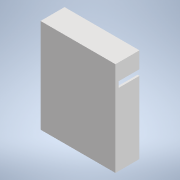
# Autodesk Inventor part: btn
Saved by Autodesk Inventor 2022 (Build 260153000, 153)
## iProperties
Created: 2025-06-23
Part Number: btn
Material: Типовые
Document SubType Name: Modeling
Designer: korsh524
Density: 1 g/cm^3
Appearance: По умолчанию
Author: korsh524
Autodesk Inventor part; units mm, degrees
ref_plane "YZ Plane" through (0, 0, 0) normal (1, 0, 0) x (0, 1, 0)
ref_plane "XZ Plane" through (0, 0, 0) normal (0, 1, 0) x (-1, 0, 0)
ref_plane "XY Plane" through (0, 0, 0) normal (0, 0, 1) x (1, 0, 0)
sketch "Эскиз1" plane through (0, 0, 0) normal (0, 0, 1) x (1, 0, 0)
  line L0 (-37, -47) -> (37, -47)
  line L1 (37, -47) -> (37, 47)
  line L2 (37, 47) -> (-37, 47)
  line L3 (-37, 47) -> (-37, -47)
  line L4 (-35, -44) -> (-35, 44) projected
  line L5 (34, -45) -> (-34, -45) projected
  line L6 (35, 44) -> (35, -44) projected
  line L7 (-34, 45) -> (34, 45) projected
  point P0 (0, 0)
  dimension "d0" = 2
  dimension "d1" = 2
  dimension "d2" = 2
  dimension "d3" = 2
  constraints: 8 end point, 2 parallel, 1 horizontal, 1 perpendicular
  measures "d0" distance between parallel lines of L3 L4
  measures "d1" distance between parallel lines of L0 L5
  measures "d2" distance between parallel lines of L6 L1
  measures "d3" distance between parallel lines of L7 L2
extrude "Выдавливание1" add sketch "Эскиз1" along normal blind 2
sketch "Эскиз2" plane through (0, 0, 2) normal (0, 0, 1) x (1, 0, 0)
  line L0 (-39, -49) -> (39, -49)
  line L1 (39, -49) -> (39, 49)
  line L2 (39, 49) -> (-39, 49)
  line L3 (-39, 49) -> (-39, -49)
  line L4 (-37, 47) -> (-37, -47) projected
  line L5 (-37, -47) -> (37, -47) projected
  line L6 (37, -47) -> (37, 47) projected
  line L7 (37, 47) -> (-37, 47) projected
  point P0 (0, 0)
  dimension "d6" = 2
  dimension "d7" = 2
  dimension "d8" = 2
  dimension "d9" = 2
  constraints: 8 end point, 2 parallel, 1 horizontal, 1 perpendicular
  measures "d6" distance between parallel lines of L3 L4
  measures "d7" distance between parallel lines of L0 L5
  measures "d8" distance between parallel lines of L6 L1
  measures "d9" distance between parallel lines of L2 L7
extrude "Выдавливание2" add sketch "Эскиз2" against normal blind 25
sketch "Эскиз3" plane through (-39, -49, 2) normal (-1, 0, 0) x (0, 0, 1)
  line L0 (-3.5, 69) -> (-3.5, 78) projected
  line L1 (-3.5, 69) -> (-14.5, 69) projected
  line L2 (-14.5, 78) -> (-14.5, 69) projected
  line L3 (-3.5, 78) -> (-14.5, 78) projected
  point P0 (-2, 49)
extrude "Выдавливание3" cut sketch "Эскиз3" against normal blind 25
sketch "Эскиз4" plane through (-39, -49, 2) normal (-1, 0, 0) x (0, 0, 1)
  line L0 (-3.5, 69) -> (-3.5, 78) projected
  line L1 (-3.5, 78) -> (-14.5, 78) projected
  line L2 (-14.5, 69) -> (-14.5, 78) projected
  line L3 (-3.5, 69) -> (-14.5, 69) projected
  line L4 (-15.0649, 68.3908) -> (-2.9071, 68.3908)
  line L5 (-2.9071, 68.3908) -> (-2.9071, 78.6857)
  line L6 (-2.9071, 78.6857) -> (-15.0649, 78.6857)
  line L7 (-15.0649, 78.6857) -> (-15.0649, 68.3908)
  point P0 (-2, 49)
  constraints: 8 end point, 2 parallel, 1 horizontal, 1 perpendicular
extrude "Выдавливание4" cut sketch "Эскиз4" against normal blind 25
sketch "Эскиз5" plane through (-39, -49, 2) normal (0, -1, 0) x (1, 0, 0)
  line L0 (19, -3.5) -> (6, -3.5) projected
  line L1 (19, -3.5) -> (19, -19.5) projected
  line L2 (6, -19.5) -> (19, -19.5) projected
  line L3 (6, -3.5) -> (6, -19.5) projected
  line L4 (65, -3.5) -> (38, -3.5) projected
  line L5 (65, -3.5) -> (65, -9.5) projected
  line L6 (54, -9.5) -> (65, -9.5) projected
  line L7 (54, -9.5) -> (54, -16.5) projected
  line L8 (38, -16.5) -> (54, -16.5) projected
  line L9 (38, -3.5) -> (38, -16.5) projected
  line L10 (2, -25) -> (76, -25) projected
  line L11 (6, -3.5) -> (54, -3.5)
  line L12 (54, -3.5) -> (54, -25)
  line L13 (54, -25) -> (6, -25)
  line L14 (6, -25) -> (6, -3.5)
  line L15 (54, -25) -> (6, -25)
  line L16 (6, -25) -> (6, -2.7247)
  line L17 (6, -2.7247) -> (54, -2.7247)
  line L18 (54, -2.7247) -> (54, -25)
  point P0 (39, -2)
  point P1 (6, -25)
  constraints: 16 end point, 4 parallel, 2 horizontal, 2 perpendicular, 1 point on line
extrude "Выдавливание5" cut sketch "Эскиз5" against normal blind 25 contours L1 L2 L3 L0 | L11 L9 L8 L12 L10 L14 L2 L1 | L4 L12 L7 L8 L9
sketch "Эскиз6" plane through (39, -49, 2) normal (1, 0, 0) x (0, 0, -1)
  arc A0 (8.5, 75) -> (8.5, 81) centre (8.5, 78) ccw projected
  arc A1 (6.5, 81) -> (6.5, 75) centre (6.5, 78) ccw projected
  line L0 (6.5, 75) -> (8.5, 75) projected
  arc A2 (8.5, 75) -> (8.5, 81) centre (8.5, 78) ccw projected
  line L1 (6.5, 81) -> (8.5, 81) projected
  line L2 (25, 0) -> (25, 98) projected
  line L3 (3.5, 81) -> (25, 81)
  line L4 (25, 81) -> (25, 75)
  line L5 (25, 75) -> (3.5, 75)
  line L6 (3.5, 75) -> (3.5, 81)
  point P0 (2, 49)
  point P1 (6.5, 75)
  point P2 (8.5, 75)
  point P3 (8.5, 81)
  point P4 (6.5, 81)
  constraints: 8 end point, 2 parallel, 1 horizontal, 1 perpendicular, 1 point on line
extrude "Выдавливание6" cut sketch "Эскиз6" against normal blind 25
sketch "Эскиз7" plane through (-39, -49, 2) normal (-1, 0, 0) x (0, 0, 1)
  point P0 (-2, 49)
sketch "Эскиз8" plane through (-39, -49, 2) normal (-1, 0, 0) x (0, 0, 1)
  line L0 (-15.0649, 68.3908) -> (-15.0649, 78.6857) projected
  line L1 (-15.0649, 78.6857) -> (-15.0649, 68.3908) projected
  line L2 (-15.0649, 68.3908) -> (-19.0649, 68.3908)
  line L3 (-19.0649, 68.3908) -> (-19.0649, 78.6857)
  line L4 (-19.0649, 78.6857) -> (-15.0649, 78.6857)
  line L5 (-15.0649, 78.6857) -> (-15.0649, 68.3908)
  point P0 (-2, 49)
  dimension "d20" = 4
  constraints: 8 end point, 2 parallel, 1 horizontal, 1 perpendicular
  measures "d20" distance of L3.end L4.end
extrude "Выдавливание7" cut sketch "Эскиз8" against normal blind 10
equation "\"d7\" = d6"
equation "\"d8\" = d7"
equation "\"d9\" = d7"
